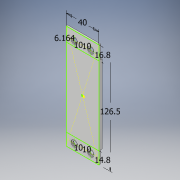
# Autodesk Inventor part: BatteryCover
Saved by Autodesk Inventor 2018 (Build 220112000, 112)
## iProperties
Created: 2017-08-07
Part Number: BatteryCover
Material: Generic
Document SubType Name: Modeling
Designer: Akram Al-Hourani
Density: 1 g/cm^3
Appearance: Default
Author: Akram Al-Hourani
Autodesk Inventor part; units mm, degrees
ref_plane "YZ Plane" through (0, 0, 0) normal (1, 0, 0) x (0, 1, 0)
ref_plane "XZ Plane" through (0, 0, 0) normal (0, 1, 0) x (-1, 0, 0)
ref_plane "XY Plane" through (0, 0, 0) normal (0, 0, 1) x (1, 0, 0)
sketch "Sketch1" plane through (0, 0, 0) normal (0, 0, 1) x (1, 0, 0)
  line L0 (-22.0545, -63.25) -> (17.9455, -63.25)
  line L1 (17.9455, -63.25) -> (17.9455, 63.25)
  line L2 (17.9455, 63.25) -> (-22.0545, 63.25)
  line L3 (-22.0545, 63.25) -> (-22.0545, -63.25)
  line L4 (-22.0545, -63.25) -> (17.9455, 63.25) construction
  line L5 (17.9455, -63.25) -> (-22.0545, 63.25) construction
  line L6 (-22.0545, -63.25) -> (17.9455, -63.25)
  line L7 (17.9455, -63.25) -> (17.9455, -48.45)
  line L8 (17.9455, -48.45) -> (-22.0545, -48.45)
  line L9 (-22.0545, -48.45) -> (-22.0545, -63.25)
  line L10 (-22.0545, -55.85) -> (17.9455, -55.85) construction
  line L11 (-2.0545, -55.85) -> (7.9455, -55.85) construction
  line L12 (-2.0545, -55.85) -> (-12.0545, -55.85) construction
  line L13 (-22.0545, 63.25) -> (17.9455, 63.25)
  line L14 (17.9455, 63.25) -> (17.9455, 46.45)
  line L15 (17.9455, 46.45) -> (-22.0545, 46.45)
  line L16 (-22.0545, 46.45) -> (-22.0545, 63.25)
  line L17 (-22.0545, 46.45) -> (-22.0545, 52.614) construction
  line L18 (-22.0545, 52.614) -> (17.9455, 52.614) construction
  line L19 (-2.0545, 52.614) -> (7.9455, 52.614) construction
  line L20 (-2.0545, 52.614) -> (-12.0545, 52.614) construction
  line L21 (-22.0545, 46.45) -> (17.9455, 46.45)
  line L22 (17.9455, 46.45) -> (17.9455, -48.45)
  line L23 (17.9455, -48.45) -> (-22.0545, -48.45)
  line L24 (-22.0545, -48.45) -> (-22.0545, 46.45)
  point P0 (0, 0)
  point P1 (-2.0545, 0)
  dimension "d0" = 40
  dimension "d1" = 126.5
  dimension "d4" = 14.8
  dimension "d5" = 10
  dimension "d6" = 10
  dimension "d9" = 16.8
  dimension "d10" = 6.164
  dimension "d11" = 10
  dimension "d12" = 10
  constraints: 50 end point, 8 parallel, 8 point on line, 6 midpoint, 5 perpendicular, 4 coincident, 4 horizontal
  measures "d0" distance of L2.end L1.end
  measures "d1" distance of L1.end L0.end
  measures "d4" distance of L7.end L6.end
  measures "d5" distance of L11.start L11.end
  measures "d6" distance of L11.start L12.end
  measures "d9" distance of L13.end L14.end
  measures "d10" distance of L15.end L17.end
  measures "d11" distance of L19.start L19.end
  measures "d12" distance of L19.start L20.end
extrude "Extrusion1" add sketch "Sketch1" against normal blind 2
extrude "Extrusion2" add sketch "Sketch1" against normal blind 4 contours L3 L15 L1 L8
hole "Hole1" at (-12.0545, 52.614, 0) at (7.9455, 52.614, 0) at (-12.0545, -55.85, 0) at (7.9455, -55.85, 0) direction (0, 0, -1) diameter 5 end through all counterbore diameter 8 counterbore depth 1
body "Solid1"
